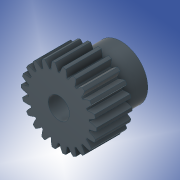
# Autodesk Inventor part: BA012
Saved by Autodesk Inventor 2017 (Build 210142000, 142)
## iProperties
Created: 2017-06-27
Part Number: BA012
Material: ABS Plastic
Document SubType Name: Modeling
Designer: zallen
Density: 1.06 g/cm^3
Appearance: CR Dark Blue
Author: zallen
Autodesk Inventor part; units mm, degrees
ref_plane "YZ Plane" through (0, 0, 0) normal (1, 0, 0) x (0, 1, 0)
ref_plane "XZ Plane" through (0, 0, 0) normal (0, 1, 0) x (-1, 0, 0)
ref_plane "XY Plane" through (0, 0, 0) normal (0, 0, 1) x (1, 0, 0)
sketch "Sketch1" plane through (0, 0, 0) normal (0, 0, 1) x (1, 0, 0)
  circle A0 centre (0, 0) radius 6
  circle A1 centre (0, 0) radius 17.25
  dimension "d0" = 12
  dimension "d1" = 34.5
  constraints: 2 centre point, 2 coincident
  measures "d0" diameter of A0
  measures "d1" diameter of A1
extrude "Extrusion1" add sketch "Sketch1" along normal blind 20
sketch "Sketch2" plane through (0, 0, 20) normal (0, 0, 1) x (1, 0, 0)
  line L0 (0, 0) -> (50.6019, 0) construction
  circle A0 centre (0, 0) radius 17.25 projected
  arc A1 (21.1337, 0.9) -> (17.1337, 2) centre (15.1945, -12.8741) ccw
  arc A2 (17.1337, -2) -> (21.1337, -0.9) centre (15.1945, 12.8741) ccw
  arc A3 (21.1337, -0.9) -> (21.1337, 0.9) centre (1.1539, 0) ccw
  arc A4 (17.1337, -2) -> (17.1337, 2) centre (0, 0) ccw
  arc A5 (20.024, 6.8176) -> (15.8762, 6.7461) centre (18.2061, -8.0718) ccw
  arc A6 (17.0031, 2.9081) -> (20.5312, 5.0905) centre (10.952, 16.6334) ccw
  arc A7 (20.5312, 5.0905) -> (20.024, 6.8176) centre (1.1072, 0.3251) ccw
  arc A8 (17.0031, 2.9081) -> (15.8762, 6.7461) centre (0, 0) ccw
  arc A9 (17.2922, 12.1829) -> (13.3325, 10.9457) centre (19.7427, -2.6156) ccw
  arc A10 (15.495, 7.5807) -> (18.2653, 10.6686) centre (5.8222, 19.0452) ccw
  arc A11 (18.2653, 10.6686) -> (17.2922, 12.1829) centre (0.9707, 0.6239) ccw
  arc A12 (15.495, 7.5807) -> (13.3325, 10.9457) centre (0, 0) ccw
  arc A13 (13.1594, 16.5611) -> (9.7087, 14.2585) centre (19.6799, 3.0525) ccw
  arc A14 (12.7317, 11.639) -> (14.5198, 15.3824) centre (0.2207, 19.914) ccw
  arc A15 (14.5198, 15.3824) -> (13.1594, 16.5611) centre (0.7557, 0.8721) ccw
  arc A16 (12.7317, 11.639) -> (9.7087, 14.2585) centre (0, 0) ccw
  arc A17 (7.9606, 19.5977) -> (5.2983, 16.4162) centre (18.0228, 8.4733) ccw
  arc A18 (8.9368, 14.7545) -> (9.5979, 18.85) centre (-5.3987, 19.1695) ccw
  arc A19 (9.5979, 18.85) -> (7.9606, 19.5977) centre (0.4794, 1.0496) ccw
  arc A20 (8.9368, 14.7545) -> (5.2983, 16.4162) centre (0, 0) ccw
  arc A21 (2.1168, 21.0466) -> (0.4587, 17.2439) centre (14.9055, 13.2077) ccw
  arc A22 (4.418, 16.6746) -> (3.8985, 20.7905) centre (-10.5807, 16.8721) ccw
  arc A23 (3.8985, 20.7905) -> (2.1168, 21.0466) centre (0.1642, 1.1422) ccw
  arc A24 (4.418, 16.6746) -> (0.4587, 17.2439) centre (0, 0) ccw
  arc A25 (-3.8985, 20.7905) -> (-4.418, 16.6746) centre (10.5807, 16.8721) ccw
  arc A26 (-0.4587, 17.2439) -> (-2.1168, 21.0466) centre (-14.9055, 13.2077) ccw
  arc A27 (-2.1168, 21.0466) -> (-3.8985, 20.7905) centre (-0.1642, 1.1422) ccw
  arc A28 (-0.4587, 17.2439) -> (-4.418, 16.6746) centre (0, 0) ccw
  arc A29 (-9.5979, 18.85) -> (-8.9368, 14.7545) centre (5.3987, 19.1695) ccw
  arc A30 (-5.2983, 16.4162) -> (-7.9606, 19.5977) centre (-18.0228, 8.4733) ccw
  arc A31 (-7.9606, 19.5977) -> (-9.5979, 18.85) centre (-0.4794, 1.0496) ccw
  arc A32 (-5.2983, 16.4162) -> (-8.9368, 14.7545) centre (0, 0) ccw
  arc A33 (-14.5198, 15.3824) -> (-12.7317, 11.639) centre (-0.2207, 19.914) ccw
  arc A34 (-9.7087, 14.2585) -> (-13.1594, 16.5611) centre (-19.6799, 3.0525) ccw
  arc A35 (-13.1594, 16.5611) -> (-14.5198, 15.3824) centre (-0.7557, 0.8721) ccw
  arc A36 (-9.7087, 14.2585) -> (-12.7317, 11.639) centre (0, 0) ccw
  arc A37 (-18.2653, 10.6686) -> (-15.495, 7.5807) centre (-5.8222, 19.0452) ccw
  arc A38 (-13.3325, 10.9457) -> (-17.2922, 12.1829) centre (-19.7427, -2.6156) ccw
  arc A39 (-17.2922, 12.1829) -> (-18.2653, 10.6686) centre (-0.9707, 0.6239) ccw
  arc A40 (-13.3325, 10.9457) -> (-15.495, 7.5807) centre (0, 0) ccw
  arc A41 (-20.5312, 5.0905) -> (-17.0031, 2.9081) centre (-10.952, 16.6334) ccw
  arc A42 (-15.8762, 6.7461) -> (-20.024, 6.8176) centre (-18.2061, -8.0718) ccw
  arc A43 (-20.024, 6.8176) -> (-20.5312, 5.0905) centre (-1.1072, 0.3251) ccw
  arc A44 (-15.8762, 6.7461) -> (-17.0031, 2.9081) centre (0, 0) ccw
  arc A45 (-21.1337, -0.9) -> (-17.1337, -2) centre (-15.1945, 12.8741) ccw
  arc A46 (-17.1337, 2) -> (-21.1337, 0.9) centre (-15.1945, -12.8741) ccw
  arc A47 (-21.1337, 0.9) -> (-21.1337, -0.9) centre (-1.1539, 0) ccw
  arc A48 (-17.1337, 2) -> (-17.1337, -2) centre (0, 0) ccw
  arc A49 (-20.024, -6.8176) -> (-15.8762, -6.7461) centre (-18.2061, 8.0718) ccw
  arc A50 (-17.0031, -2.9081) -> (-20.5312, -5.0905) centre (-10.952, -16.6334) ccw
  arc A51 (-20.5312, -5.0905) -> (-20.024, -6.8176) centre (-1.1072, -0.3251) ccw
  arc A52 (-17.0031, -2.9081) -> (-15.8762, -6.7461) centre (0, 0) ccw
  arc A53 (-17.2922, -12.1829) -> (-13.3325, -10.9457) centre (-19.7427, 2.6156) ccw
  arc A54 (-15.495, -7.5807) -> (-18.2653, -10.6686) centre (-5.8222, -19.0452) ccw
  arc A55 (-18.2653, -10.6686) -> (-17.2922, -12.1829) centre (-0.9707, -0.6239) ccw
  arc A56 (-15.495, -7.5807) -> (-13.3325, -10.9457) centre (0, 0) ccw
  arc A57 (-13.1594, -16.5611) -> (-9.7087, -14.2585) centre (-19.6799, -3.0525) ccw
  arc A58 (-12.7317, -11.639) -> (-14.5198, -15.3824) centre (-0.2207, -19.914) ccw
  arc A59 (-14.5198, -15.3824) -> (-13.1594, -16.5611) centre (-0.7557, -0.8721) ccw
  arc A60 (-12.7317, -11.639) -> (-9.7087, -14.2585) centre (0, 0) ccw
  arc A61 (-7.9606, -19.5977) -> (-5.2983, -16.4162) centre (-18.0228, -8.4733) ccw
  arc A62 (-8.9368, -14.7545) -> (-9.5979, -18.85) centre (5.3987, -19.1695) ccw
  arc A63 (-9.5979, -18.85) -> (-7.9606, -19.5977) centre (-0.4794, -1.0496) ccw
  arc A64 (-8.9368, -14.7545) -> (-5.2983, -16.4162) centre (0, 0) ccw
  arc A65 (-2.1168, -21.0466) -> (-0.4587, -17.2439) centre (-14.9055, -13.2077) ccw
  arc A66 (-4.418, -16.6746) -> (-3.8985, -20.7905) centre (10.5807, -16.8721) ccw
  arc A67 (-3.8985, -20.7905) -> (-2.1168, -21.0466) centre (-0.1642, -1.1422) ccw
  arc A68 (-4.418, -16.6746) -> (-0.4587, -17.2439) centre (0, 0) ccw
  arc A69 (3.8985, -20.7905) -> (4.418, -16.6746) centre (-10.5807, -16.8721) ccw
  arc A70 (0.4587, -17.2439) -> (2.1168, -21.0466) centre (14.9055, -13.2077) ccw
  arc A71 (2.1168, -21.0466) -> (3.8985, -20.7905) centre (0.1642, -1.1422) ccw
  arc A72 (0.4587, -17.2439) -> (4.418, -16.6746) centre (0, 0) ccw
  arc A73 (9.5979, -18.85) -> (8.9368, -14.7545) centre (-5.3987, -19.1695) ccw
  arc A74 (5.2983, -16.4162) -> (7.9606, -19.5977) centre (18.0228, -8.4733) ccw
  arc A75 (7.9606, -19.5977) -> (9.5979, -18.85) centre (0.4794, -1.0496) ccw
  arc A76 (5.2983, -16.4162) -> (8.9368, -14.7545) centre (0, 0) ccw
  arc A77 (14.5198, -15.3824) -> (12.7317, -11.639) centre (0.2207, -19.914) ccw
  arc A78 (9.7087, -14.2585) -> (13.1594, -16.5611) centre (19.6799, -3.0525) ccw
  arc A79 (13.1594, -16.5611) -> (14.5198, -15.3824) centre (0.7557, -0.8721) ccw
  arc A80 (9.7087, -14.2585) -> (12.7317, -11.639) centre (0, 0) ccw
  arc A81 (18.2653, -10.6686) -> (15.495, -7.5807) centre (5.8222, -19.0452) ccw
  arc A82 (13.3325, -10.9457) -> (17.2922, -12.1829) centre (19.7427, 2.6156) ccw
  arc A83 (17.2922, -12.1829) -> (18.2653, -10.6686) centre (0.9707, -0.6239) ccw
  arc A84 (13.3325, -10.9457) -> (15.495, -7.5807) centre (0, 0) ccw
  arc A85 (20.5312, -5.0905) -> (17.0031, -2.9081) centre (10.952, -16.6334) ccw
  arc A86 (15.8762, -6.7461) -> (20.024, -6.8176) centre (18.2061, 8.0718) ccw
  arc A87 (20.024, -6.8176) -> (20.5312, -5.0905) centre (1.1072, -0.3251) ccw
  arc A88 (15.8762, -6.7461) -> (17.0031, -2.9081) centre (0, 0) ccw
  point P0 (21.1539, 0)
  point P1 (20.297, 5.9597)
  point P2 (17.7958, 11.4367)
  point P3 (13.8529, 15.9871)
  point P4 (8.7877, 19.2423)
  point P5 (3.0105, 20.9386)
  point P6 (-3.0105, 20.9386)
  point P7 (-8.7877, 19.2423)
  point P8 (-13.8529, 15.9871)
  point P9 (-17.7958, 11.4367)
  point P10 (-20.297, 5.9597)
  point P11 (-21.1539, 0)
  point P12 (-20.297, -5.9597)
  point P13 (-17.7958, -11.4367)
  point P14 (-13.8529, -15.9871)
  point P15 (-8.7877, -19.2423)
  point P16 (-3.0105, -20.9386)
  point P17 (3.0105, -20.9386)
  point P18 (8.7877, -19.2423)
  point P19 (13.8529, -15.9871)
  point P20 (17.7958, -11.4367)
  point P21 (20.297, -5.9597)
  dimension "d4" = 15
  dimension "d5" = 15
  dimension "d6" = 20
  dimension "d7" = 4
  dimension "d8" = 1.8
  dimension "d9" = 2
  dimension "d12" = 360
  constraints: 179 point on circle, 88 centre point, 2 end point, 2 vertical alignment, 1 concentric, 1 horizontal, 1 point on line, 287 other
  measures "d4" radius of A1
  measures "d5" radius of A2
  measures "d6" radius of A3
  measures "d7" horizontal distance of A1.start A0.start
  measures "d8" distance of A2.end A1.start
  measures "d9" distance from line of L0 A0.start
extrude "Extrusion2" add sketch "Sketch2" against normal blind 20 contours A0 A1 A3 A2 | A0 A5 A7 A6 | A85 A87 A86 A0 | A0 A9 A11 A10 | A81 A83 A82 A0 | A0 A13 A15 A14 | A77 A79 A78 A0 | A0 A17 A19 A18 | A73 A75 A74 A0 | A0 A21 A23 A22 | A69 A71 A70 A0 | A0 A25 A27 A26 | A65 A67 A66 A0 | A0 A29 A31 A30 | A61 A63 A62 A0 | A0 A33 A35 A34 | A57 A59 A58 A0 | A0 A37 A39 A38 | A53 A55 A54 A0 | A0 A41 A43 A42 | A49 A51 A50 A0 | A0 A45 A47 A46
sketch "Sketch3" plane through (0, 0, 0) normal (0, 0, -1) x (-1, 0, 0)
  circle A0 centre (0, 0) radius 6 projected
  circle A1 centre (0, 0) radius 15
  dimension "d16" = 30
  constraints: 1 centre point, 1 coincident
  measures "d16" diameter of A1
extrude "Extrusion3" add sketch "Sketch3" along normal blind 15
body "Solid1"
